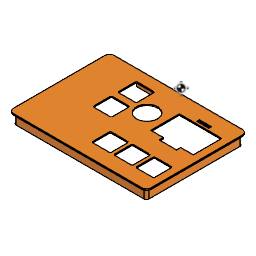
Carcasa y botones (Autodesk Fusion 360 design; units mm, degrees)
Autodesk Fusion 360 part; units mm, degrees
note: some values were not read from the file. Chosen so that the rebuilt part matches the saved one: which bodies a step acts on. Set by a fixed rule: which sketch regions a step uses.
(part 1 of 2)
sketch "Boceto1" plane through (0, 0, 0) normal (0, 0, 1) x (1, 0, 0)
  line L0 (-2, 76) -> (102, 76)
  line L1 (106, 72) -> (106, -2)
  line L2 (102, -6) -> (-2, -6)
  line L3 (-6, -2) -> (-6, 72)
  arc A0 (102, -6) -> (106, -2) centre (102, -2) ccw
  arc A1 (106, 72) -> (102, 76) centre (102, 72) ccw
  arc A2 (-2, 76) -> (-6, 72) centre (-2, 72) ccw
  arc A3 (-6, -2) -> (-2, -6) centre (-2, -2) ccw
  line L4 (-2, 72) -> (102, 72)
  line L5 (-2, -2) -> (-2, 72)
  line L6 (102, -2) -> (-2, -2)
  line L7 (102, 72) -> (102, -2)
  line L8 (0, 0) -> (100, 0)
  line L9 (100, 0) -> (100, 70)
  line L10 (100, 70) -> (0, 70)
  line L11 (0, 70) -> (0, 0)
  circle A4 centre (1.8, 68) radius 0.75
  circle A5 centre (1.8, 68) radius 1.25
  circle A6 centre (1.8, 2) radius 0.75
  circle A7 centre (48.2, 68) radius 0.75
  circle A8 centre (48.2, 68) radius 1.25
  circle A9 centre (1.8, 2) radius 1.25
  circle A10 centre (48.2, 2) radius 1.5
  circle A11 centre (48.2, 2) radius 1
  circle A12 centre (98.2, 2) radius 1.5
  circle A13 centre (98.2, 2) radius 1
  circle A14 centre (51.8, 2) radius 0.75
  circle A15 centre (51.8, 2) radius 1.25
  circle A16 centre (51.8, 68) radius 1.25
  circle A17 centre (51.8, 68) radius 0.75
  circle A18 centre (98.2, 68) radius 0.75
  circle A19 centre (98.2, 68) radius 1.25
  arc A20 (-2, 74) -> (-4, 72) centre (-2, 72) ccw
  line L12 (-4, -2) -> (-4, 72)
  arc A21 (-4, -2) -> (-2, -4) centre (-2, -2) ccw
  line L13 (102, -4) -> (-2, -4)
  arc A22 (102, -4) -> (104, -2) centre (102, -2) ccw
  line L14 (104, 72) -> (104, -2)
  arc A23 (104, 72) -> (102, 74) centre (102, 72) ccw
  line L15 (-2, 74) -> (102, 74)
  point P0 (-6, 76)
  point P1 (106, 76)
  point P2 (-6, -6)
  point P3 (50, 70)
  point P4 (50, 70)
  dimension "d23" = 50
  dimension "d29" = 4
  dimension "d30" = 4
  dimension "d31" = 4
  dimension "d32" = 4
  dimension "d35" = 4
  dimension "d173" = 0
  dimension "d194" = 15
  dimension "d199" = 1
  dimension "d282" = 50
  dimension "d285" = 100
  dimension "d286" = 70
  dimension "d287" = 1.5
  dimension "d288" = 0.5
  dimension "d289" = 1.5
  dimension "d290" = 66
  dimension "d291" = 1.5
  dimension "d292" = 46.4
  dimension "d293" = 2
  dimension "d294" = 1.8
  dimension "d295" = 0.5
  dimension "d296" = 0.5
  dimension "d297" = 2
  dimension "d298" = 1.8
  dimension "d303" = 2
  dimension "d306" = 50
  dimension "d307" = 0
  dimension "d308" = 1.8
  dimension "d321" = 2
  dimension "d322" = 2
  dimension "d323" = -2
  dimension "d335" = 6
  dimension "d336" = 6
  dimension "d363" = 50
  dimension "d398" = 15
  dimension "d399" = 15
  dimension "d472" = 2.54
  dimension "d557" = 1
  dimension "d592" = 1
  constraint horizontal L0
  constraint vertical L1
  constraint horizontal L2
  constraint vertical L3
  constraint tangent L1 A0
  constraint tangent L2 A0
  constraint coincident P1 L0
  constraint coincident P1 L1
  constraint tangent L0 A1
  constraint tangent L1 A1
  constraint coincident P0 L0
  constraint coincident P0 L3
  constraint tangent L0 A2
  constraint tangent L3 A2
  constraint coincident P2 L2
  constraint coincident P2 L3
  constraint tangent L2 A3
  constraint tangent L3 A3
  constraint horizontal L8
  constraint vertical L9
  constraint horizontal L10
  constraint vertical L11
  constraint coincident L8.start L11.end
  constraint midpoint L10 P4
  measures "d29" radius of A0
  measures "d30" radius of A1
  measures "d31" radius of A2
  measures "d32" radius of A3
  measures "d285" distance of L8.start L8.end
  measures "d286" distance of L8.start L10.end
  measures "d287" diameter of A4
  measures "d289" diameter of A6
  measures "d290" vertical distance of A4.centre A6.centre
  measures "d291" diameter of A7
  measures "d292" horizontal distance of A4.centre A7.centre
  measures "d293" distance of L10 A4.centre
  measures "d294" distance of L11 A4.centre
  measures "d297" distance of L8 A6.centre
  measures "d298" horizontal distance of A7.centre P4
  measures "d303" distance of L10 A7.centre
  measures "d308" distance of L11 A6.centre
  measures "d321" distance of L5 L11
  measures "d322" distance of L4 L10
  measures "d335" distance of L3 L10.end
  measures "d336" distance of L0 L10.end
extrude "Extruir10" add sketch "Boceto1" along normal blind 2 contours L8 L9 L10 L11 | A4 | A5 | A6 | A7 | A8 | A9 | A10 | A11 | A12 | A13 | A14 | A15 | A16 | A17 | A18 | A19 makes body 1
extrude "Extruir41" add sketch "Boceto1" along normal blind 5 separate body contours A5 makes body 2
extrude "Extruir42" add sketch "Boceto1" along normal blind 6 contours A4 bodies 2
pattern_linear "Patrón R4" count 2 spacing 66 along (0, -1, 0) count 2 spacing 46.4 along (1, 0, 0) of bodies 2 makes body 3 at (3.0484, 1.9377, 3.3333) makes body 4 at (49.4113, 68.3084, 3.3333) makes body 5 at (49.4484, 1.9377, 3.3333)
pattern_linear "Patrón R5" count 2 spacing 50 along (1, 0, 0) of bodies 2 3 4 5 makes body 6 at (53.0113, 68.3084, 3.3333) makes body 7 at (53.0484, 1.9377, 3.3333) makes body 8 at (98.5386, 69.2033, 3.3333) makes body 9 at (98.5386, 3.2033, 3.3333)
combine "Combinar3" operation add target body 1 tool bodies 6 3 4 5 7 9 8 2
extrude "Extruir13" add sketch "Boceto1" along normal blind 2 contours L4 L5 L6 L7 bodies 1
extrude "Extruir14" add sketch "Boceto1" along normal blind 28 contours L0 L1 L2 L3 A0 A1 A2 A3 | A20 L12 A21 L13 A22 L14 A23 L15 bodies 1
sketch "Boceto4" plane through (0, 0, 28) normal (0, 0, 1) x (-1, 0, 0)
  line L0 (2, -72) -> (-102, -72)
  line L1 (-102, -72) -> (-102, 2)
  line L2 (-102, 2) -> (2, 2)
  line L3 (2, 2) -> (2, -72)
  arc A0 (2, -76) -> (6, -72) centre (2, -72) ccw
  line L4 (6, -72) -> (6, 2)
  arc A1 (6, 2) -> (2, 6) centre (2, 2) ccw
  line L5 (2, 6) -> (-102, 6)
  arc A2 (-102, 6) -> (-106, 2) centre (-102, 2) ccw
  line L6 (-106, 2) -> (-106, -72)
  arc A3 (-106, -72) -> (-102, -76) centre (-102, -72) ccw
  line L7 (-102, -76) -> (2, -76)
  line L8 (2, 6) -> (-102, 6)
  arc A4 (-102, 6) -> (-106, 2) centre (-102, 2) ccw
  line L9 (-106, 2) -> (-106, -72)
  arc A5 (-106, -72) -> (-102, -76) centre (-102, -72) ccw
  line L10 (-102, -76) -> (2, -76)
  arc A6 (2, -76) -> (6, -72) centre (2, -72) ccw
  line L11 (6, -72) -> (6, 2)
  arc A7 (6, 2) -> (2, 6) centre (2, 2) ccw
  line L12 (2, 4) -> (-102, 4)
  arc A8 (-102, 4) -> (-104, 2) centre (-102, 2) ccw
  line L13 (-104, 2) -> (-104, -72)
  arc A9 (-104, -72) -> (-102, -74) centre (-102, -72) ccw
  line L14 (-102, -74) -> (2, -74)
  arc A10 (2, -74) -> (4, -72) centre (2, -72) ccw
  line L15 (4, -72) -> (4, 2)
  arc A11 (4, 2) -> (2, 4) centre (2, 2) ccw
  dimension "d328" = -2
extrude "Extruir16" cut sketch "Boceto4" against normal blind 8 contours L12 A8 L13 A9 L14 A10 L15 A11 bodies 1
extrude "Extruir17" add sketch "Boceto4" along normal blind 8 separate body contours A0 L4 A1 L5 A2 L6 A3 L7 L8 A4 L9 A5 L10 A6 L11 A7 | L12 A8 L13 A9 L14 A10 L15 A11 makes body 10
extrude "Extruir18" add sketch "Boceto4" along normal blind 9 contours L0 L1 L2 L3 | A0 L4 A1 L5 A2 L6 A3 L7 L8 A4 L9 A5 L10 A6 L11 A7 | L12 A8 L13 A9 L14 A10 L15 A11 bodies 10
extrude "Extruir19" cut sketch "Boceto4" along normal blind 8 bodies 10
extrude "Extruir21" add sketch "Boceto4" along normal blind 9 contours L0 L1 L2 L3 bodies 10
extrude "Extruir22" cut sketch "Boceto4" along normal blind 8 contours L0 L1 L2 L3 bodies 10
move_body "Desplazar1" bodies 10 to x (1, 0, 0) y (0, 1, 0) z (0, 0, 1) at (115, 0, 0)
sketch "Boceto5" plane through (0, 0, 37) normal (0, 0, 1) x (-1, 0, 0)
  line L0 (-217, -76) -> (-113, -76)
  arc A0 (-113, -76) -> (-109, -72) centre (-113, -72) ccw
  line L1 (-109, -72) -> (-109, 2)
  arc A1 (-109, 2) -> (-113, 6) centre (-113, 2) ccw
  line L2 (-113, 6) -> (-217, 6)
  arc A2 (-217, 6) -> (-221, 2) centre (-217, 2) ccw
  line L3 (-221, 2) -> (-221, -72)
  arc A3 (-221, -72) -> (-217, -76) centre (-217, -72) ccw
  line L4 (-179.92, -66.21) -> (-215.32, -66.21)
  line L5 (-215.32, -66.21) -> (-215.32, -32.86)
  line L6 (-215.32, -32.86) -> (-179.92, -32.86)
  line L7 (-179.92, -32.86) -> (-179.92, -66.21)
  circle A4 centre (-182.42, -63.71) radius 1.675
  line L8 (-197.62, -66.21) -> (-197.62, -32.86)
  circle A5 centre (-212.82, -63.71) radius 1.675
  line L9 (-179.92, -49.535) -> (-215.32, -49.535)
  circle A6 centre (-182.42, -35.36) radius 1.675
  circle A7 centre (-212.82, -35.36) radius 1.675
  line L10 (-180.445, -61.21) -> (-214.845, -61.21)
  line L11 (-214.845, -61.21) -> (-214.845, -38.21)
  line L12 (-214.845, -38.21) -> (-180.445, -38.21)
  line L13 (-180.445, -38.21) -> (-180.445, -61.21)
  circle A8 centre (-166.49, -48.97) radius 7.5
  circle A9 centre (-166.49, -48.97) radius 8.5
  line L14 (-115, -70) -> (-215, -70)
  line L15 (-215, -70) -> (-215, 0)
  line L16 (-215, 0) -> (-115, 0)
  line L17 (-115, 0) -> (-115, -70)
  arc A10 (-196.5, -5.91) -> (-197.5, -6.9059) centre (-196.5, -6.91) ccw
  line L18 (-183.5, -20.91) -> (-196.5001, -20.91)
  line L19 (-197.5, -19.8978) -> (-197.5, -6.9059)
  line L20 (-182.5, -6.91) -> (-182.5, -19.91)
  line L21 (-196.5, -5.91) -> (-183.5, -5.91)
  arc A11 (-197.5, -19.8978) -> (-196.5001, -20.91) centre (-196.5001, -19.91) ccw
  arc A12 (-182.5, -6.91) -> (-183.5, -5.91) centre (-183.5, -6.91) ccw
  arc A13 (-183.5, -20.91) -> (-182.5, -19.91) centre (-183.5, -19.91) ccw
  line L22 (-118.41, -64.21) -> (-136.19, -64.21)
  line L23 (-136.19, -64.21) -> (-136.19, -5.79)
  line L24 (-136.19, -5.79) -> (-118.41, -5.79)
  line L25 (-118.41, -5.79) -> (-118.41, -64.21)
  line L26 (-154.12, -51.63) -> (-141.12, -51.63)
  arc A14 (-154.12, -51.63) -> (-155.12, -52.6246) centre (-154.12, -52.63) ccw
  line L27 (-155.12, -65.6161) -> (-155.12, -52.6246)
  line L28 (-140.12, -52.63) -> (-140.12, -65.63)
  arc A15 (-155.12, -65.6161) -> (-154.1201, -66.63) centre (-154.1201, -65.63) ccw
  arc A16 (-140.12, -52.63) -> (-141.12, -51.63) centre (-141.12, -52.63) ccw
  arc A17 (-141.12, -66.63) -> (-140.12, -65.63) centre (-141.12, -65.63) ccw
  line L29 (-141.12, -66.63) -> (-154.1201, -66.63)
  line L30 (-214.28, -5.91) -> (-201.28, -5.91)
  arc A18 (-214.28, -5.91) -> (-215.28, -6.9057) centre (-214.28, -6.91) ccw
  line L31 (-215.28, -19.8963) -> (-215.28, -6.9057)
  arc A19 (-200.28, -6.91) -> (-201.28, -5.91) centre (-201.28, -6.91) ccw
  line L32 (-201.28, -20.91) -> (-214.2801, -20.91)
  line L33 (-200.28, -6.91) -> (-200.28, -19.91)
  arc A20 (-215.28, -19.8963) -> (-214.2801, -20.91) centre (-214.2801, -19.91) ccw
  arc A21 (-201.28, -20.91) -> (-200.28, -19.91) centre (-201.28, -19.91) ccw
  line L34 (-154.12, -31.31) -> (-141.12, -31.31)
  arc A22 (-154.12, -31.31) -> (-155.12, -32.3051) centre (-154.12, -32.31) ccw
  line L35 (-155.12, -45.2969) -> (-155.12, -32.3051)
  arc A23 (-140.12, -32.31) -> (-141.12, -31.31) centre (-141.12, -32.31) ccw
  line L36 (-141.12, -46.31) -> (-154.1201, -46.31)
  line L37 (-140.12, -32.31) -> (-140.12, -45.31)
  arc A24 (-155.12, -45.2969) -> (-154.1201, -46.31) centre (-154.1201, -45.31) ccw
  arc A25 (-141.12, -46.31) -> (-140.12, -45.31) centre (-141.12, -45.31) ccw
  line L38 (-178.72, -5.91) -> (-165.72, -5.91)
  arc A26 (-178.72, -5.91) -> (-179.72, -6.9059) centre (-178.72, -6.91) ccw
  line L39 (-179.72, -19.8979) -> (-179.72, -6.9059)
  arc A27 (-164.72, -6.91) -> (-165.72, -5.91) centre (-165.72, -6.91) ccw
  line L40 (-165.72, -20.91) -> (-178.7201, -20.91)
  line L41 (-164.72, -6.91) -> (-164.72, -19.91)
  arc A28 (-179.72, -19.8979) -> (-178.7201, -20.91) centre (-178.7201, -19.91) ccw
  arc A29 (-165.72, -20.91) -> (-164.72, -19.91) centre (-165.72, -19.91) ccw
  line L42 (-190.62, -38.21) -> (-190.62, -34.86)
  line L43 (-190.62, -34.86) -> (-197.62, -34.86)
  line L44 (-204.62, -38.21) -> (-204.62, -34.86)
  line L45 (-204.62, -34.86) -> (-197.62, -34.86)
  circle A30 centre (-193.81, -64.21) radius 1
  line L46 (-192.81, -65.21) -> (-197.62, -65.21)
  line L47 (-197.62, -65.21) -> (-197.62, -63.21)
  line L48 (-197.62, -63.21) -> (-192.81, -63.21)
  line L49 (-192.81, -63.21) -> (-192.81, -65.21)
  line L50 (-202.43, -65.21) -> (-197.62, -65.21)
  line L51 (-202.43, -63.21) -> (-202.43, -65.21)
  line L52 (-197.62, -63.21) -> (-202.43, -63.21)
  point P0 (-118.41, -64.21)
  point P1 (-120.95, -64.21)
  point P2 (-123.49, -64.21)
  point P3 (-126.03, -64.21)
  point P4 (-128.57, -64.21)
  point P5 (-131.11, -64.21)
  point P6 (-133.65, -64.21)
  point P7 (-136.19, -64.21)
  point P8 (-138.73, -64.21)
  point P9 (-141.27, -64.21)
  point P10 (-143.81, -64.21)
  point P11 (-146.35, -64.21)
  point P12 (-148.89, -64.21)
  point P13 (-151.43, -64.21)
  point P14 (-153.97, -64.21)
  point P15 (-156.51, -64.21)
  point P16 (-159.05, -64.21)
  point P17 (-161.59, -64.21)
  point P18 (-118.41, -61.67)
  point P19 (-120.95, -61.67)
  point P20 (-123.49, -61.67)
  point P21 (-126.03, -61.67)
  point P22 (-128.57, -61.67)
  point P23 (-131.11, -61.67)
  point P24 (-133.65, -61.67)
  point P25 (-136.19, -61.67)
  point P26 (-138.73, -61.67)
  point P27 (-141.27, -61.67)
  point P28 (-143.81, -61.67)
  point P29 (-146.35, -61.67)
  point P30 (-148.89, -61.67)
  point P31 (-151.43, -61.67)
  point P32 (-153.97, -61.67)
  point P33 (-156.51, -61.67)
  point P34 (-159.05, -61.67)
  point P35 (-161.59, -61.67)
  point P36 (-118.41, -59.13)
  point P37 (-120.95, -59.13)
  point P38 (-123.49, -59.13)
  point P39 (-126.03, -59.13)
  point P40 (-128.57, -59.13)
  point P41 (-131.11, -59.13)
  point P42 (-133.65, -59.13)
  point P43 (-136.19, -59.13)
  point P44 (-138.73, -59.13)
  point P45 (-141.27, -59.13)
  point P46 (-143.81, -59.13)
  point P47 (-146.35, -59.13)
  point P48 (-148.89, -59.13)
  point P49 (-151.43, -59.13)
  point P50 (-153.97, -59.13)
  point P51 (-156.51, -59.13)
  point P52 (-159.05, -59.13)
  point P53 (-161.59, -59.13)
  point P54 (-118.41, -56.59)
  point P55 (-120.95, -56.59)
  point P56 (-123.49, -56.59)
  point P57 (-126.03, -56.59)
  point P58 (-128.57, -56.59)
  point P59 (-131.11, -56.59)
  point P60 (-133.65, -56.59)
  point P61 (-136.19, -56.59)
  point P62 (-138.73, -56.59)
  point P63 (-141.27, -56.59)
  point P64 (-143.81, -56.59)
  point P65 (-146.35, -56.59)
  point P66 (-148.89, -56.59)
  point P67 (-151.43, -56.59)
  point P68 (-153.97, -56.59)
  point P69 (-156.51, -56.59)
  point P70 (-159.05, -56.59)
  point P71 (-161.59, -56.59)
  point P72 (-118.41, -54.05)
  point P73 (-120.95, -54.05)
  point P74 (-123.49, -54.05)
  point P75 (-126.03, -54.05)
  point P76 (-128.57, -54.05)
  point P77 (-131.11, -54.05)
  point P78 (-133.65, -54.05)
  point P79 (-136.19, -54.05)
  point P80 (-138.73, -54.05)
  point P81 (-141.27, -54.05)
  point P82 (-143.81, -54.05)
  point P83 (-146.35, -54.05)
  point P84 (-148.89, -54.05)
  point P85 (-151.43, -54.05)
  point P86 (-153.97, -54.05)
  point P87 (-156.51, -54.05)
  point P88 (-159.05, -54.05)
  point P89 (-161.59, -54.05)
  point P90 (-118.41, -51.51)
  point P91 (-120.95, -51.51)
  point P92 (-123.49, -51.51)
  point P93 (-126.03, -51.51)
  point P94 (-128.57, -51.51)
  point P95 (-131.11, -51.51)
  point P96 (-133.65, -51.51)
  point P97 (-136.19, -51.51)
  point P98 (-138.73, -51.51)
  point P99 (-141.27, -51.51)
  point P100 (-143.81, -51.51)
  point P101 (-146.35, -51.51)
  point P102 (-148.89, -51.51)
  point P103 (-151.43, -51.51)
  point P104 (-153.97, -51.51)
  point P105 (-156.51, -51.51)
  point P106 (-159.05, -51.51)
  point P107 (-161.59, -51.51)
  point P108 (-118.41, -48.97)
  point P109 (-120.95, -48.97)
  point P110 (-123.49, -48.97)
  point P111 (-126.03, -48.97)
  point P112 (-128.57, -48.97)
  point P113 (-131.11, -48.97)
  point P114 (-133.65, -48.97)
  point P115 (-136.19, -48.97)
  point P116 (-138.73, -48.97)
  point P117 (-141.27, -48.97)
  point P118 (-143.81, -48.97)
  point P119 (-146.35, -48.97)
  point P120 (-148.89, -48.97)
  point P121 (-151.43, -48.97)
  point P122 (-153.97, -48.97)
  point P123 (-156.51, -48.97)
  point P124 (-159.05, -48.97)
  point P125 (-161.59, -48.97)
  point P126 (-118.41, -46.43)
  point P127 (-120.95, -46.43)
  point P128 (-123.49, -46.43)
  point P129 (-126.03, -46.43)
  point P130 (-128.57, -46.43)
  point P131 (-131.11, -46.43)
  point P132 (-133.65, -46.43)
  point P133 (-136.19, -46.43)
  point P134 (-138.73, -46.43)
  point P135 (-141.27, -46.43)
  point P136 (-143.81, -46.43)
  point P137 (-146.35, -46.43)
  point P138 (-148.89, -46.43)
  point P139 (-151.43, -46.43)
  point P140 (-153.97, -46.43)
  point P141 (-156.51, -46.43)
  point P142 (-159.05, -46.43)
  point P143 (-161.59, -46.43)
  point P144 (-118.41, -43.89)
  point P145 (-120.95, -43.89)
  point P146 (-123.49, -43.89)
  point P147 (-126.03, -43.89)
  point P148 (-128.57, -43.89)
  point P149 (-131.11, -43.89)
  point P150 (-133.65, -43.89)
  point P151 (-136.19, -43.89)
  point P152 (-138.73, -43.89)
  point P153 (-141.27, -43.89)
  point P154 (-143.81, -43.89)
  point P155 (-146.35, -43.89)
  point P156 (-148.89, -43.89)
  point P157 (-151.43, -43.89)
  point P158 (-153.97, -43.89)
  point P159 (-156.51, -43.89)
  point P160 (-159.05, -43.89)
  point P161 (-161.59, -43.89)
  point P162 (-118.41, -41.35)
  point P163 (-120.95, -41.35)
  point P164 (-123.49, -41.35)
  point P165 (-126.03, -41.35)
  point P166 (-128.57, -41.35)
  point P167 (-131.11, -41.35)
  point P168 (-133.65, -41.35)
  point P169 (-136.19, -41.35)
  point P170 (-138.73, -41.35)
  point P171 (-141.27, -41.35)
  point P172 (-143.81, -41.35)
  point P173 (-146.35, -41.35)
  point P174 (-148.89, -41.35)
  point P175 (-151.43, -41.35)
  point P176 (-153.97, -41.35)
  point P177 (-156.51, -41.35)
  point P178 (-159.05, -41.35)
  point P179 (-161.59, -41.35)
  point P180 (-118.41, -38.81)
  point P181 (-120.95, -38.81)
  point P182 (-123.49, -38.81)
  point P183 (-126.03, -38.81)
  point P184 (-128.57, -38.81)
  point P185 (-131.11, -38.81)
  point P186 (-133.65, -38.81)
  point P187 (-136.19, -38.81)
  point P188 (-138.73, -38.81)
  point P189 (-141.27, -38.81)
  point P190 (-143.81, -38.81)
  point P191 (-146.35, -38.81)
  point P192 (-148.89, -38.81)
  point P193 (-151.43, -38.81)
  point P194 (-153.97, -38.81)
  point P195 (-156.51, -38.81)
  point P196 (-159.05, -38.81)
  point P197 (-161.59, -38.81)
  point P198 (-118.41, -36.27)
  point P199 (-120.95, -36.27)
  point P200 (-123.49, -36.27)
  point P201 (-126.03, -36.27)
  point P202 (-128.57, -36.27)
  point P203 (-131.11, -36.27)
  point P204 (-133.65, -36.27)
  point P205 (-136.19, -36.27)
  point P206 (-138.73, -36.27)
  point P207 (-141.27, -36.27)
  point P208 (-143.81, -36.27)
  point P209 (-146.35, -36.27)
  point P210 (-148.89, -36.27)
  point P211 (-151.43, -36.27)
  point P212 (-153.97, -36.27)
  point P213 (-156.51, -36.27)
  point P214 (-159.05, -36.27)
  point P215 (-161.59, -36.27)
  point P216 (-118.41, -33.73)
  point P217 (-120.95, -33.73)
  point P218 (-123.49, -33.73)
  point P219 (-126.03, -33.73)
  point P220 (-128.57, -33.73)
  point P221 (-131.11, -33.73)
  point P222 (-133.65, -33.73)
  point P223 (-136.19, -33.73)
  point P224 (-138.73, -33.73)
  point P225 (-141.27, -33.73)
  point P226 (-143.81, -33.73)
  point P227 (-146.35, -33.73)
  point P228 (-148.89, -33.73)
  point P229 (-151.43, -33.73)
  point P230 (-153.97, -33.73)
  point P231 (-156.51, -33.73)
  point P232 (-159.05, -33.73)
  point P233 (-161.59, -33.73)
  point P234 (-118.41, -31.19)
  point P235 (-120.95, -31.19)
  point P236 (-123.49, -31.19)
  point P237 (-126.03, -31.19)
  point P238 (-128.57, -31.19)
  point P239 (-131.11, -31.19)
  point P240 (-133.65, -31.19)
  point P241 (-136.19, -31.19)
  point P242 (-138.73, -31.19)
  point P243 (-141.27, -31.19)
  point P244 (-143.81, -31.19)
  point P245 (-146.35, -31.19)
  point P246 (-148.89, -31.19)
  point P247 (-151.43, -31.19)
  point P248 (-153.97, -31.19)
  point P249 (-156.51, -31.19)
  point P250 (-159.05, -31.19)
  point P251 (-161.59, -31.19)
  point P252 (-118.41, -28.65)
  point P253 (-120.95, -28.65)
  point P254 (-123.49, -28.65)
  point P255 (-126.03, -28.65)
  point P256 (-128.57, -28.65)
  point P257 (-131.11, -28.65)
  point P258 (-133.65, -28.65)
  point P259 (-136.19, -28.65)
  point P260 (-138.73, -28.65)
  point P261 (-141.27, -28.65)
  point P262 (-143.81, -28.65)
  point P263 (-146.35, -28.65)
  point P264 (-148.89, -28.65)
  point P265 (-151.43, -28.65)
  point P266 (-153.97, -28.65)
  point P267 (-156.51, -28.65)
  point P268 (-159.05, -28.65)
  point P269 (-161.59, -28.65)
  point P270 (-118.41, -26.11)
  point P271 (-120.95, -26.11)
  point P272 (-123.49, -26.11)
  point P273 (-126.03, -26.11)
  point P274 (-128.57, -26.11)
  point P275 (-131.11, -26.11)
  point P276 (-133.65, -26.11)
  point P277 (-136.19, -26.11)
  point P278 (-138.73, -26.11)
  point P279 (-141.27, -26.11)
  point P280 (-143.81, -26.11)
  point P281 (-146.35, -26.11)
  point P282 (-148.89, -26.11)
  point P283 (-151.43, -26.11)
  point P284 (-153.97, -26.11)
  point P285 (-156.51, -26.11)
  point P286 (-159.05, -26.11)
  point P287 (-161.59, -26.11)
  point P288 (-118.41, -23.57)
  point P289 (-120.95, -23.57)
  point P290 (-123.49, -23.57)
  point P291 (-126.03, -23.57)
  point P292 (-128.57, -23.57)
  point P293 (-131.11, -23.57)
  point P294 (-133.65, -23.57)
  point P295 (-136.19, -23.57)
  point P296 (-138.73, -23.57)
  point P297 (-141.27, -23.57)
  point P298 (-143.81, -23.57)
  point P299 (-146.35, -23.57)
  point P300 (-148.89, -23.57)
  point P301 (-151.43, -23.57)
  point P302 (-153.97, -23.57)
  point P303 (-156.51, -23.57)
  point P304 (-159.05, -23.57)
  point P305 (-161.59, -23.57)
  point P306 (-118.41, -21.03)
  point P307 (-120.95, -21.03)
  point P308 (-123.49, -21.03)
  point P309 (-126.03, -21.03)
  point P310 (-128.57, -21.03)
  point P311 (-131.11, -21.03)
  point P312 (-133.65, -21.03)
  point P313 (-136.19, -21.03)
  point P314 (-138.73, -21.03)
  point P315 (-141.27, -21.03)
  point P316 (-143.81, -21.03)
  point P317 (-146.35, -21.03)
  point P318 (-148.89, -21.03)
  point P319 (-151.43, -21.03)
  point P320 (-153.97, -21.03)
  point P321 (-156.51, -21.03)
  point P322 (-159.05, -21.03)
  point P323 (-161.59, -21.03)
  point P324 (-118.41, -18.49)
  point P325 (-120.95, -18.49)
  point P326 (-123.49, -18.49)
  point P327 (-126.03, -18.49)
  point P328 (-128.57, -18.49)
  point P329 (-131.11, -18.49)
  point P330 (-133.65, -18.49)
  point P331 (-136.19, -18.49)
  point P332 (-138.73, -18.49)
  point P333 (-141.27, -18.49)
  point P334 (-143.81, -18.49)
  point P335 (-146.35, -18.49)
  point P336 (-148.89, -18.49)
  point P337 (-151.43, -18.49)
  point P338 (-153.97, -18.49)
  point P339 (-156.51, -18.49)
  point P340 (-159.05, -18.49)
  point P341 (-161.59, -18.49)
  point P342 (-118.41, -15.95)
  point P343 (-120.95, -15.95)
  point P344 (-123.49, -15.95)
  point P345 (-126.03, -15.95)
  point P346 (-128.57, -15.95)
  point P347 (-131.11, -15.95)
  point P348 (-133.65, -15.95)
  point P349 (-136.19, -15.95)
  point P350 (-138.73, -15.95)
  point P351 (-141.27, -15.95)
  point P352 (-143.81, -15.95)
  point P353 (-146.35, -15.95)
  point P354 (-148.89, -15.95)
  point P355 (-151.43, -15.95)
  point P356 (-153.97, -15.95)
  point P357 (-156.51, -15.95)
  point P358 (-159.05, -15.95)
  point P359 (-161.59, -15.95)
  point P360 (-118.41, -13.41)
  point P361 (-120.95, -13.41)
  point P362 (-123.49, -13.41)
  point P363 (-126.03, -13.41)
  point P364 (-128.57, -13.41)
  point P365 (-131.11, -13.41)
  point P366 (-133.65, -13.41)
  point P367 (-136.19, -13.41)
  point P368 (-138.73, -13.41)
  point P369 (-141.27, -13.41)
  point P370 (-143.81, -13.41)
  point P371 (-146.35, -13.41)
  point P372 (-148.89, -13.41)
  point P373 (-151.43, -13.41)
  point P374 (-153.97, -13.41)
  point P375 (-156.51, -13.41)
  point P376 (-159.05, -13.41)
  point P377 (-161.59, -13.41)
  point P378 (-118.41, -10.87)
  point P379 (-120.95, -10.87)
  point P380 (-123.49, -10.87)
  point P381 (-126.03, -10.87)
  point P382 (-128.57, -10.87)
  point P383 (-131.11, -10.87)
  point P384 (-133.65, -10.87)
  point P385 (-136.19, -10.87)
  point P386 (-138.73, -10.87)
  point P387 (-141.27, -10.87)
  point P388 (-143.81, -10.87)
  point P389 (-146.35, -10.87)
  point P390 (-148.89, -10.87)
  point P391 (-151.43, -10.87)
  point P392 (-153.97, -10.87)
  point P393 (-156.51, -10.87)
  point P394 (-159.05, -10.87)
  point P395 (-161.59, -10.87)
  point P396 (-118.41, -8.33)
  point P397 (-120.95, -8.33)
  point P398 (-123.49, -8.33)
  point P399 (-126.03, -8.33)
  point P400 (-128.57, -8.33)
  point P401 (-131.11, -8.33)
  point P402 (-133.65, -8.33)
  point P403 (-136.19, -8.33)
  point P404 (-138.73, -8.33)
  point P405 (-141.27, -8.33)
  point P406 (-143.81, -8.33)
  point P407 (-146.35, -8.33)
  point P408 (-148.89, -8.33)
  point P409 (-151.43, -8.33)
  point P410 (-153.97, -8.33)
  point P411 (-156.51, -8.33)
  point P412 (-159.05, -8.33)
  point P413 (-161.59, -8.33)
  point P414 (-118.41, -5.79)
  point P415 (-120.95, -5.79)
  point P416 (-123.49, -5.79)
  point P417 (-126.03, -5.79)
  point P418 (-128.57, -5.79)
  point P419 (-131.11, -5.79)
  point P420 (-133.65, -5.79)
  point P421 (-136.19, -5.79)
  point P422 (-138.73, -5.79)
  point P423 (-141.27, -5.79)
  point P424 (-143.81, -5.79)
  point P425 (-146.35, -5.79)
  point P426 (-148.89, -5.79)
  point P427 (-151.43, -5.79)
  point P428 (-153.97, -5.79)
  point P429 (-156.51, -5.79)
  point P430 (-159.05, -5.79)
  point P431 (-161.59, -5.79)
  point P432 (-188.73, -46.43)
  point P433 (-186.19, -46.43)
  point P434 (-170.95, -31.19)
  point P435 (-193.81, -41.35)
  point P436 (-209.05, -26.11)
  point P437 (-198.89, -48.97)
  point P438 (-196.35, -48.97)
  point P439 (-201.43, -26.11)
  point P440 (-206.51, -26.11)
  point P441 (-170.95, -26.11)
  point P442 (-181.11, -31.19)
  point P443 (-183.65, -28.65)
  point P444 (-183.65, -31.19)
  point P445 (-198.89, -41.35)
  point P446 (-191.27, -43.89)
  point P447 (-196.35, -46.43)
  point P448 (-188.73, -48.97)
  point P449 (-188.73, -31.19)
  point P450 (-168.41, -26.11)
  point P451 (-196.35, -43.89)
  point P452 (-193.81, -48.97)
  point P453 (-188.73, -26.11)
  point P454 (-191.27, -48.97)
  point P455 (-193.81, -46.43)
  point P456 (-198.89, -43.89)
  point P457 (-203.97, -31.19)
  point P458 (-193.81, -28.65)
  point P459 (-203.97, -28.65)
  point P460 (-191.27, -46.43)
  point P461 (-188.73, -43.89)
  point P462 (-191.27, -31.19)
  point P463 (-193.81, -43.89)
  point P464 (-196.35, -41.35)
  point P465 (-206.51, -28.65)
  point P466 (-188.73, -41.35)
  point P467 (-201.43, -28.65)
  point P468 (-198.89, -46.43)
  point P469 (-196.35, -31.19)
  point P470 (-203.97, -46.43)
  point P471 (-191.27, -41.35)
  point P472 (-209.05, -43.89)
  point P473 (-198.89, -31.19)
  point P474 (-198.89, -28.65)
  point P475 (-191.27, -26.11)
  point P476 (-211.59, -28.65)
  point P477 (-206.51, -48.97)
  point P478 (-209.05, -31.19)
  point P479 (-206.51, -41.35)
  point P480 (-193.81, -31.19)
  point P481 (-211.59, -48.97)
  point P482 (-211.59, -41.35)
  point P483 (-211.59, -31.19)
  point P484 (-196.35, -26.11)
  point P485 (-203.97, -48.97)
  point P486 (-196.35, -28.65)
  point P487 (-211.59, -26.11)
  point P488 (-209.05, -48.97)
  point P489 (-188.73, -28.65)
  point P490 (-209.05, -46.43)
  point P491 (-206.51, -43.89)
  point P492 (-191.27, -28.65)
  point P493 (-201.43, -31.19)
  point P494 (-198.89, -26.11)
  point P495 (-209.05, -41.35)
  point P496 (-193.81, -26.11)
  point P497 (-206.51, -46.43)
  point P498 (-203.97, -43.89)
  point P499 (-201.43, -46.43)
  point P500 (-211.59, -46.43)
  point P501 (-203.97, -26.11)
  point P502 (-209.05, -28.65)
  point P503 (-206.51, -31.19)
  point P504 (-203.97, -41.35)
  point P505 (-201.43, -41.35)
  point P506 (-201.43, -43.89)
  point P507 (-168.41, -18.49)
  point P508 (-170.95, -23.57)
  point P509 (-211.59, -43.89)
  point P510 (-168.41, -21.03)
  point P511 (-183.65, -38.81)
  point P512 (-168.41, -36.27)
  point P513 (-186.19, -38.81)
  point P514 (-183.65, -21.03)
  point P515 (-186.19, -23.57)
  point P516 (-176.03, -21.03)
  point P517 (-178.57, -18.49)
  point P518 (-201.43, -48.97)
  point P519 (-170.95, -51.51)
  point P520 (-170.95, -33.73)
  point P521 (-173.49, -38.81)
  point P522 (-181.11, -51.51)
  point P523 (-181.11, -36.27)
  point P524 (-173.49, -23.57)
  point P525 (-173.49, -54.05)
  point P526 (-170.95, -21.03)
  point P527 (-186.19, -33.73)
  point P528 (-170.95, -38.81)
  point P529 (-176.03, -51.51)
  point P530 (-173.49, -21.03)
  point P531 (-183.65, -54.05)
  point P532 (-176.03, -54.05)
  point P533 (-181.11, -56.59)
  point P534 (-181.11, -21.03)
  point P535 (-168.41, -33.73)
  point P536 (-178.57, -36.27)
  point P537 (-186.19, -21.03)
  point P538 (-181.11, -54.05)
  point P539 (-181.11, -33.73)
  point P540 (-176.03, -56.59)
  point P541 (-181.11, -23.57)
  point P542 (-176.03, -18.49)
  point P543 (-183.65, -33.73)
  point P544 (-176.03, -33.73)
  point P545 (-176.03, -23.57)
  point P546 (-178.57, -21.03)
  point P547 (-186.19, -56.59)
  point P548 (-186.19, -54.05)
  point P549 (-168.41, -51.51)
  point P550 (-170.95, -18.49)
  point P551 (-178.57, -33.73)
  point P552 (-173.49, -18.49)
  point P553 (-170.95, -36.27)
  point P554 (-186.19, -51.51)
  point P555 (-178.57, -51.51)
  point P556 (-183.65, -23.57)
  point P557 (-181.11, -38.81)
  point P558 (-173.49, -56.59)
  point P559 (-186.19, -36.27)
  point P560 (-183.65, -56.59)
  point P561 (-176.03, -38.81)
  point P562 (-183.65, -18.49)
  point P563 (-168.41, -38.81)
  point P564 (-181.11, -18.49)
  point P565 (-173.49, -51.51)
  point P566 (-173.49, -33.73)
  point P567 (-168.41, -23.57)
  point P568 (-170.95, -56.59)
  point P569 (-211.59, -21.03)
  point P570 (-183.65, -51.51)
  point P571 (-168.41, -54.05)
  point P572 (-170.95, -54.05)
  point P573 (-193.81, -23.57)
  point P574 (-173.49, -36.27)
  point P575 (-178.57, -23.57)
  point P576 (-183.65, -36.27)
  point P577 (-186.19, -18.49)
  point P578 (-176.03, -36.27)
  point P579 (-168.41, -56.59)
  point P580 (-178.57, -56.59)
  point P581 (-211.59, -33.73)
  point P582 (-191.27, -36.27)
  point P583 (-178.57, -54.05)
  point P584 (-178.57, -38.81)
  point P585 (-191.27, -18.49)
  point P586 (-206.51, -23.57)
  point P587 (-201.43, -36.27)
  point P588 (-196.35, -23.57)
  point P589 (-203.97, -23.57)
  point P590 (-211.59, -18.49)
  point P591 (-198.89, -33.73)
  point P592 (-206.51, -51.51)
  point P593 (-211.59, -23.57)
  point P594 (-209.05, -54.05)
  point P595 (-193.81, -33.73)
  point P596 (-211.59, -38.81)
  point P597 (-173.49, -64.21)
  point P598 (-206.51, -18.49)
  point P599 (-206.51, -56.59)
  point P600 (-203.97, -36.27)
  point P601 (-188.73, -38.81)
  point P602 (-176.03, -61.67)
  point P603 (-168.41, -61.67)
  point P604 (-196.35, -21.03)
  point P605 (-196.35, -18.49)
  point P606 (-188.73, -51.51)
  point P607 (-201.43, -38.81)
  point P608 (-176.03, -64.21)
  point P609 (-193.81, -36.27)
  point P610 (-188.73, -54.05)
  point P611 (-203.97, -54.05)
  point P612 (-186.19, -61.67)
  point P613 (-201.43, -23.57)
  point P614 (-188.73, -36.27)
  point P615 (-198.89, -51.51)
  point P616 (-203.97, -21.03)
  point P617 (-209.05, -21.03)
  point P618 (-209.05, -23.57)
  point P619 (-181.11, -61.67)
  point P620 (-196.35, -33.73)
  point P621 (-198.89, -21.03)
  point P622 (-206.51, -36.27)
  point P623 (-209.05, -51.51)
  point P624 (-203.97, -33.73)
  point P625 (-191.27, -51.51)
  point P626 (-188.73, -18.49)
  point P627 (-173.49, -59.13)
  point P628 (-206.51, -38.81)
  point P629 (-193.81, -18.49)
  point P630 (-193.81, -56.59)
  point P631 (-203.97, -18.49)
  point P632 (-196.35, -38.81)
  point P633 (-209.05, -33.73)
  point P634 (-170.95, -64.21)
  point P635 (-201.43, -21.03)
  point P636 (-193.81, -51.51)
  point P637 (-211.59, -51.51)
  point P638 (-191.27, -23.57)
  point P639 (-191.27, -33.73)
  point P640 (-188.73, -33.73)
  point P641 (-188.73, -21.03)
  point P642 (-173.49, -61.67)
  point P643 (-191.27, -38.81)
  point P644 (-191.27, -21.03)
  point P645 (-178.57, -59.13)
  point P646 (-211.59, -36.27)
  point P647 (-211.59, -54.05)
  point P648 (-196.35, -54.05)
  point P649 (-186.19, -59.13)
  point P650 (-193.81, -38.81)
  point P651 (-201.43, -51.51)
  point P652 (-183.65, -64.21)
  point P653 (-193.81, -21.03)
  point P654 (-178.57, -64.21)
  point P655 (-209.05, -56.59)
  point P656 (-198.89, -18.49)
  point P657 (-203.97, -51.51)
  point P658 (-201.43, -18.49)
  point P659 (-206.51, -33.73)
  point P660 (-178.57, -61.67)
  point P661 (-198.89, -38.81)
  point P662 (-196.35, -56.59)
  point P663 (-201.43, -33.73)
  point P664 (-188.73, -23.57)
  point P665 (-209.05, -18.49)
  point P666 (-196.35, -51.51)
  point P667 (-183.65, -61.67)
  point P668 (-198.89, -36.27)
  point P669 (-183.65, -59.13)
  point P670 (-209.05, -38.81)
  point P671 (-209.05, -36.27)
  point P672 (-198.89, -56.59)
  point P673 (-168.41, -59.13)
  point P674 (-196.35, -36.27)
  point P675 (-170.95, -61.67)
  point P676 (-198.89, -23.57)
  point P677 (-211.59, -56.59)
  point P678 (-201.43, -56.59)
  point P679 (-201.43, -54.05)
  point P680 (-206.51, -21.03)
  point P681 (-188.73, -56.59)
  point P682 (-168.41, -64.21)
  point P683 (-181.11, -64.21)
  point P684 (-186.19, -64.21)
  point P685 (-191.27, -56.59)
  point P686 (-198.89, -54.05)
  point P687 (-203.97, -38.81)
  point P688 (-206.51, -54.05)
  point P689 (-191.27, -54.05)
  point P690 (-198.89, -59.13)
  point P691 (-193.81, -54.05)
  point P692 (-176.03, -59.13)
  point P693 (-209.05, -64.21)
  point P694 (-188.73, -64.21)
  point P695 (-191.27, -61.67)
  point P696 (-203.97, -56.59)
  point P697 (-188.73, -59.13)
  point P698 (-196.35, -64.21)
  point P699 (-198.89, -64.21)
  point P700 (-193.81, -59.13)
  point P701 (-201.43, -64.21)
  point P702 (-211.59, -59.13)
  point P703 (-206.51, -61.67)
  point P704 (-191.27, -59.13)
  point P705 (-193.81, -61.67)
  point P706 (-203.97, -64.21)
  point P707 (-188.73, -61.67)
  point P708 (-196.35, -59.13)
  point P709 (-211.59, -64.21)
  point P710 (-170.95, -59.13)
  point P711 (-209.05, -61.67)
  point P712 (-191.27, -64.21)
  point P713 (-203.97, -61.67)
  point P714 (-193.81, -64.21)
  point P715 (-209.05, -59.13)
  point P716 (-181.11, -59.13)
  point P717 (-206.51, -59.13)
  point P718 (-203.97, -59.13)
  point P719 (-196.35, -61.67)
  point P720 (-201.43, -61.67)
  point P721 (-198.89, -61.67)
  point P722 (-201.43, -59.13)
  point P723 (-173.49, -41.35)
  point P724 (-173.49, -48.97)
  point P725 (-168.41, -41.35)
  point P726 (-186.19, -43.89)
  point P727 (-186.19, -41.35)
  point P728 (-183.65, -48.97)
  point P729 (-173.49, -28.65)
  point P730 (-178.57, -46.43)
  point P731 (-181.11, -28.65)
  point P732 (-183.65, -26.11)
  point P733 (-170.95, -48.97)
  point P734 (-186.19, -26.11)
  point P735 (-170.95, -41.35)
  point P736 (-186.19, -48.97)
  point P737 (-178.57, -41.35)
  point P738 (-170.95, -46.43)
  point P739 (-170.95, -43.89)
  point P740 (-183.65, -41.35)
  point P741 (-178.57, -43.89)
  point P742 (-181.11, -46.43)
  point P743 (-173.49, -43.89)
  point P744 (-176.03, -43.89)
  point P745 (-181.11, -43.89)
  point P746 (-168.41, -28.65)
  point P747 (-178.57, -28.65)
  point P748 (-168.41, -43.89)
  point P749 (-181.11, -48.97)
  point P750 (-181.11, -41.35)
  point P751 (-176.03, -46.43)
  point P752 (-178.57, -26.11)
  point P753 (-173.49, -31.19)
  point P754 (-186.19, -31.19)
  point P755 (-168.41, -48.97)
  point P756 (-176.03, -48.97)
  point P757 (-170.95, -28.65)
  point P758 (-178.57, -48.97)
  point P759 (-168.41, -46.43)
  point P760 (-176.03, -41.35)
  point P761 (-173.49, -26.11)
  point P762 (-178.57, -31.19)
  point P763 (-186.19, -28.65)
  point P764 (-181.11, -26.11)
  point P765 (-183.65, -43.89)
  point P766 (-176.03, -31.19)
  point P767 (-176.03, -28.65)
  point P768 (-173.49, -46.43)
  point P769 (-168.41, -31.19)
  point P770 (-183.65, -46.43)
  point P771 (-176.03, -26.11)
  point P772 (-211.59, -61.67)
  point P773 (-206.51, -64.21)
  point P774 (-190, -13.41)
  point P775 (-182.5, -5.91)
  point P776 (-197.5, -20.91)
  point P777 (-190, -13.41)
  point P778 (-193.81, -15.95)
  point P779 (-182.5, -20.91)
  point P780 (-173.49, -51.51)
  point P781 (-158.99, -48.97)
  point P782 (-173.49, -46.43)
  point P783 (-158.99, -51.51)
  point P784 (-158.99, -46.43)
  point P785 (-193.81, -64.21)
  point P786 (-196.35, -64.21)
  point P787 (-198.89, -64.21)
  point P788 (-201.43, -64.21)
  point P789 (-151.43, -61.67)
  point P790 (-155.12, -66.63)
  point P791 (-140.12, -66.63)
  point P792 (-147.62, -59.13)
  point P793 (-140.12, -51.63)
  point P794 (-147.62, -59.13)
  point P795 (-178.57, -10.87)
  point P796 (-209.05, -13.41)
  point P797 (-201.43, -15.95)
  point P798 (-203.97, -10.87)
  point P799 (-206.51, -15.95)
  point P800 (-203.97, -5.79)
  point P801 (-196.35, -13.41)
  point P802 (-211.59, -13.41)
  point P803 (-196.35, -15.95)
  point P804 (-186.19, -13.41)
  point P805 (-183.65, -15.95)
  point P806 (-191.27, -13.41)
  point P807 (-198.89, -13.41)
  point P808 (-203.97, -13.41)
  point P809 (-198.89, -5.79)
  point P810 (-186.19, -5.79)
  point P811 (-188.73, -8.33)
  point P812 (-186.19, -8.33)
  point P813 (-201.43, -10.87)
  point P814 (-201.43, -5.79)
  point P815 (-183.65, -10.87)
  point P816 (-206.51, -8.33)
  point P817 (-206.51, -10.87)
  point P818 (-196.35, -10.87)
  point P819 (-193.81, -8.33)
  point P820 (-183.65, -5.79)
  point P821 (-196.35, -8.33)
  point P822 (-209.05, -8.33)
  point P823 (-173.49, -15.95)
  point P824 (-170.95, -15.95)
  point P825 (-170.95, -10.87)
  point P826 (-168.41, -15.95)
  point P827 (-176.03, -15.95)
  point P828 (-173.49, -8.33)
  point P829 (-203.97, -8.33)
  point P830 (-201.43, -8.33)
  point P831 (-209.05, -5.79)
  point P832 (-191.27, -10.87)
  point P833 (-188.73, -10.87)
  point P834 (-178.57, -13.41)
  point P835 (-209.05, -10.87)
  point P836 (-211.59, -10.87)
  point P837 (-191.27, -8.33)
  point P838 (-211.59, -8.33)
  point P839 (-186.19, -10.87)
  point P840 (-193.81, -10.87)
  point P841 (-178.57, -15.95)
  point P842 (-173.49, -10.87)
  point P843 (-168.41, -13.41)
  point P844 (-176.03, -5.79)
  point P845 (-170.95, -13.41)
  point P846 (-173.49, -5.79)
  point P847 (-176.03, -10.87)
  point P848 (-168.41, -5.79)
  point P849 (-170.95, -8.33)
  point P850 (-176.03, -13.41)
  point P851 (-168.41, -8.33)
  point P852 (-176.03, -8.33)
  point P853 (-168.41, -10.87)
  point P854 (-170.95, -5.79)
  point P855 (-173.49, -13.41)
  point P856 (-196.35, -5.79)
  point P857 (-178.57, -8.33)
  point P858 (-198.89, -8.33)
  point P859 (-181.11, -5.79)
  point P860 (-181.11, -8.33)
  point P861 (-191.27, -5.79)
  point P862 (-193.81, -5.79)
  point P863 (-183.65, -8.33)
  point P864 (-211.59, -5.79)
  point P865 (-181.11, -10.87)
  point P866 (-206.51, -5.79)
  point P867 (-188.73, -5.79)
  point P868 (-178.57, -5.79)
  point P869 (-206.51, -13.41)
  point P870 (-209.05, -15.95)
  point P871 (-211.59, -15.95)
  point P872 (-198.89, -10.87)
  point P873 (-183.65, -13.41)
  point P874 (-188.73, -13.41)
  point P875 (-203.97, -15.95)
  point P876 (-181.11, -15.95)
  point P877 (-181.11, -13.41)
  point P878 (-191.27, -15.95)
  point P879 (-198.89, -15.95)
  point P880 (-201.43, -13.41)
  point P881 (-193.81, -15.95)
  point P882 (-188.73, -15.95)
  point P883 (-193.81, -13.41)
  point P884 (-186.19, -15.95)
  point P885 (-207.78, -13.41)
  point P886 (-215.28, -20.91)
  point P887 (-211.59, -15.95)
  point P888 (-200.28, -20.91)
  point P889 (-200.28, -5.91)
  point P890 (-207.78, -13.41)
  point P891 (-147.62, -38.81)
  point P892 (-155.12, -46.31)
  point P893 (-151.43, -41.35)
  point P894 (-140.12, -46.31)
  point P895 (-140.12, -31.31)
  point P896 (-147.62, -38.81)
  point P897 (-172.22, -13.41)
  point P898 (-179.72, -20.91)
  point P899 (-176.03, -15.95)
  point P900 (-164.72, -20.91)
  point P901 (-164.72, -5.91)
  point P902 (-172.22, -13.41)
  dimension "d125" = 35.4
  dimension "d126" = 33.35
  dimension "d127" = 3.35
  dimension "d131" = 2.5
  dimension "d132" = 2.5
  dimension "d133" = 34.4
  dimension "d134" = 23
  dimension "d135" = 2.5
  dimension "d136" = 0.475
  dimension "d141" = 15
  dimension "d142" = 1
  dimension "d339" = 100
  dimension "d341" = 70
  dimension "d342" = 6
  dimension "d343" = 6
  dimension "d385" = -43.18
  dimension "d386" = 58.42
  dimension "d387" = 3.41
  dimension "d388" = 43.18
  dimension "d389" = 58.42
  dimension "d390" = 5.79
  dimension "d436" = 15
  dimension "d437" = 15
  dimension "d438" = 1
  dimension "d439" = 7.5
  dimension "d440" = 7.5
  dimension "d441" = 3.81
  dimension "d442" = 2.54
  dimension "d443" = 5.08
  dimension "d444" = 2.54
  dimension "d445" = 2.54
  dimension "d446" = 2.54
  dimension "d447" = 7.5
  dimension "d448" = 7
  dimension "d449" = 7
  dimension "d450" = 7.5
  dimension "d451" = 7.5
  dimension "d452" = 2.54
  dimension "d453" = 2.54
  dimension "d454" = 13.89
  dimension "d455" = 2.54
  dimension "d458" = 3.81
  dimension "d460" = 2.54
  dimension "d461" = 2.54
  dimension "d462" = 2
  dimension "d463" = 2
  dimension "d464" = 15
  dimension "d465" = 15
  dimension "d466" = 1
  dimension "d467" = 7.5
  dimension "d468" = 7.5
  dimension "d469" = 3.81
  dimension "d470" = 2.54
  dimension "d473" = 15
  dimension "d474" = 15
  dimension "d475" = 1
  dimension "d476" = 7.5
  dimension "d477" = 7.5
  dimension "d478" = 3.81
  dimension "d479" = 2.54
  dimension "d480" = 15
  dimension "d481" = 15
  dimension "d482" = 1
  dimension "d483" = 7.5
  dimension "d484" = 7.5
  dimension "d485" = 3.81
  dimension "d486" = 2.54
  dimension "d487" = 15
  dimension "d488" = 15
  dimension "d489" = 1
  dimension "d490" = 7.5
  dimension "d491" = 7.5
  dimension "d492" = 3.81
  dimension "d493" = 2.54
  dimension "d603" = 3.35
  dimension "d604" = 7
  dimension "d608" = 2
  constraint horizontal L4
  constraint vertical L5
  constraint horizontal L6
  constraint vertical L7
  constraint midpoint L4 L8.start
  constraint midpoint L6 L8.end
  constraint symmetric A4 L8 A5
  constraint midpoint L7 L9.start
  constraint midpoint L5 L9.end
  constraint symmetric A4 L9 A6
  constraint symmetric A5 L9 A7
  constraint horizontal L10
  constraint vertical L11
  constraint horizontal L12
  constraint vertical L13
  constraint horizontal L14
  constraint vertical L15
  constraint vertical L17
  constraint horizontal L18
  constraint vertical L19
  constraint horizontal L21
  constraint vertical L20
  constraint coincident P779 L18
  constraint coincident P779 L20
  constraint tangent L18 A13
  constraint tangent L20 A13
  constraint coincident P776 L18
  constraint coincident P776 L19
  constraint tangent L18 A11
  constraint equal A11 A13
  constraint tangent A10 L21
  constraint equal A10 A13
  constraint coincident P775 L21
  constraint coincident P775 L20
  constraint tangent L21 A12
  constraint tangent L20 A12
  constraint equal A12 A13
  constraint coincident P777 P774
  constraint collinear P785 P786 P787
  constraint collinear P786 P787 P788
  constraint horizontal L22
  constraint vertical L23
  constraint horizontal L24
  constraint vertical L25
  constraint coincident P421 L23.end
  constraint coincident P0 L22.start
  constraint horizontal L29
  constraint vertical L27
  constraint horizontal L26
  constraint vertical L28
  constraint coincident P791 L29
  constraint coincident P791 L28
  constraint tangent A17 L29
  constraint tangent L28 A17
  constraint coincident P790 L29
  constraint coincident P790 L27
  constraint tangent A15 L29
  constraint equal A15 A17
  constraint tangent L26 A14
  constraint equal A14 A17
  constraint coincident P793 L26
  constraint coincident P793 L28
  constraint tangent L26 A16
  constraint tangent L28 A16
  constraint equal A16 A17
  constraint coincident P794 P792
  constraint horizontal L32
  constraint vertical L31
  constraint horizontal L30
  constraint vertical L33
  constraint coincident P888 L32
  constraint coincident P888 L33
  constraint tangent L32 A21
  constraint tangent L33 A21
  constraint coincident P886 L32
  constraint coincident P886 L31
  constraint tangent L32 A20
  constraint equal A20 A21
  constraint tangent L30 A18
  constraint equal A18 A21
  constraint coincident P889 L30
  constraint coincident P889 L33
  constraint tangent L30 A19
  constraint tangent A19 L33
  constraint equal A19 A21
  constraint coincident P890 P885
  constraint horizontal L36
  constraint vertical L35
  constraint horizontal L34
  constraint vertical L37
  constraint coincident P894 L36
  constraint coincident P894 L37
  constraint tangent L36 A25
  constraint tangent L37 A25
  constraint coincident P892 L36
  constraint coincident P892 L35
  constraint tangent L36 A24
  constraint equal A24 A25
  constraint tangent L34 A22
  constraint equal A22 A25
  constraint coincident P895 L34
  constraint coincident P895 L37
  constraint tangent L34 A23
  constraint tangent A23 L37
  constraint equal A23 A25
  constraint coincident P896 P891
  constraint horizontal L40
  constraint vertical L39
  constraint horizontal L38
  constraint vertical L41
  constraint coincident P900 L40
  constraint coincident P900 L41
  constraint tangent L40 A29
  constraint tangent L41 A29
  constraint coincident P898 L40
  constraint coincident P898 L39
  constraint tangent L40 A28
  constraint equal A28 A29
  constraint tangent L38 A26
  constraint equal A26 A29
  constraint coincident P901 L38
  constraint coincident P901 L41
  constraint tangent L38 A27
  constraint tangent A27 L41
  constraint equal A27 A29
  constraint coincident P902 P897
  constraint coincident P893 P175
  constraint coincident P780 P565
  constraint coincident P789 P31
  constraint coincident P787 P699
  constraint coincident P899 P827
  constraint coincident P881 P778
  constraint coincident P887 P871
  constraint coincident L12 L42.start
  constraint perpendicular L12 L42
  constraint coincident L8 L43.end
  constraint perpendicular L8 L43
  constraint symmetric L8 L42.start L44.start
  constraint symmetric L8 L42.end L44.end
  constraint symmetric L8 L43.end L45.end
  constraint coincident P785 P714
  constraint horizontal L46
  constraint vertical L47
  constraint horizontal L48
  constraint vertical L49
  constraint coincident L8 L47.end
  constraint tangent A30 L46
  constraint tangent A30 L48
  constraint tangent A30 L49
  constraint symmetric L8 L46.start L50.start
  constraint symmetric L8 L46.end L47.start
  constraint symmetric L8 L47.end L48.start
  constraint symmetric L8 L48.end L51.start
  measures "d125" distance of L4.start L4.end
  measures "d126" distance of L4.start L6.end
  measures "d127" diameter of A4
  measures "d131" horizontal distance of L4.start A4.centre
  measures "d132" vertical distance of L4.start A4.centre
  measures "d133" distance of L10.start L10.end
  measures "d134" distance of L10.start L12.end
  measures "d135" distance of A4.centre L10
  measures "d136" distance of L5 L11
  measures "d141" diameter of A8
  measures "d339" distance of L15.end L16.end
  measures "d341" distance of L14.end L15.end
  measures "d342" distance of L1 L14.start
  measures "d343" distance of L0 L14
  measures "d387" distance of L17 P0
  measures "d388" distance of P0 P17
  measures "d389" distance of P0 P414
  measures "d390" distance of L14 P0
  measures "d436" distance of P775 P779
  measures "d437" distance of P776 P779
  measures "d438" radius of A13
  measures "d439" distance of P777 L21
  measures "d440" distance of P777 L19
  measures "d441" horizontal distance of P777 P881
  measures "d442" vertical distance of P777 P881
  measures "d443" distance of P780 P782
  measures "d444" distance of P0 P1
  measures "d445" distance of P781 P783
  measures "d446" distance of P781 P784
  measures "d447" horizontal distance of A8.centre P783
  measures "d448" horizontal distance of A8.centre P780
  measures "d449" horizontal distance of A8.centre P782
  measures "d450" horizontal distance of A8.centre P784
  measures "d451" horizontal distance of A8.centre P781
  measures "d452" vertical distance of A8.centre P784
  measures "d453" vertical distance of A8.centre P780
  measures "d454" distance of L7 P785
  measures "d455" horizontal distance of P785 P786
  measures "d458" distance of L8 P785
  measures "d460" horizontal distance of P786 P787
  measures "d461" horizontal distance of P787 P788
  measures "d462" distance of L4 P785
  measures "d463" distance of L4 P788
  measures "d464" distance of P791 P793
  measures "d465" distance of P790 P791
  measures "d466" radius of A17
  measures "d467" distance of P794 L26
  measures "d468" distance of P794 L27
  measures "d469" horizontal distance of P789 P794
  measures "d470" vertical distance of P789 P794
  measures "d473" distance of P888 P889
  measures "d474" distance of P886 P888
  measures "d475" radius of A21
  measures "d476" distance of P890 L30
  measures "d477" distance of P890 L31
  measures "d478" horizontal distance of P887 P890
  measures "d479" vertical distance of P887 P890
  measures "d480" distance of P894 P895
  measures "d481" distance of P892 P894
  measures "d482" radius of A25
  measures "d483" distance of P896 L34
  measures "d484" distance of P896 L35
  measures "d485" horizontal distance of P893 P896
  measures "d486" vertical distance of P893 P896